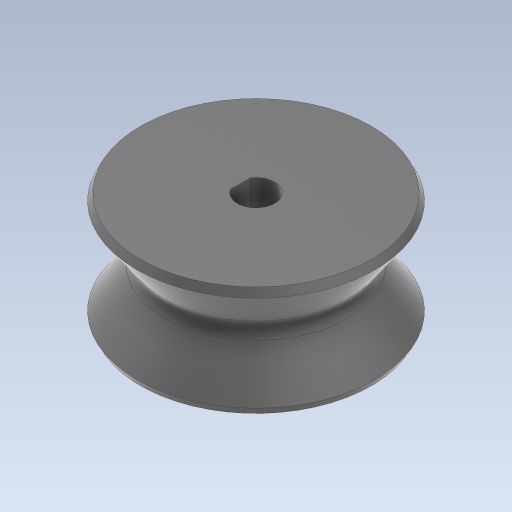
# Autodesk Inventor part: Stepper Pulley V12
Saved by Autodesk Inventor 2023 (Build 270158000, 158)
## iProperties
Created: 2022-07-02
Part Number: Stepper Pulley V12
Material: Thermoplastic Resin
Document SubType Name: Modeling
Designer: david
Density: 1.28 g/cm^3
Appearance: Smooth - Black
Author: david
## iProperties of the stored document Stepper Pulley V12_3DPrint.ipt
Created: 2022-11-09
Part Number: Stepper Pulley V12_3DPrint
Material: Generic
Document SubType Name: Modeling
Designer: Dave
Density: 1 g/cm^3
Appearance: Default
Author: Dave
Autodesk Inventor part; units mm, degrees
ref_plane "YZ Plane" through (0, 0, 0) normal (1, 0, 0) x (0, 1, 0)
sketch "Sketch1" plane through (0, 0, 0) normal (0, 1, 0) x (-1, 0, 0)
  arc A0 (2.15, 1.3711) -> (2.15, -1.3711) centre (0, 0) ccw
  line L0 (2.15, 1.3711) -> (2.15, -1.3711)
  dimension "d1" = 4.7
  dimension "d92" = 2.55
  constraints: 2 end point, 2 point on circle, 1 centre point, 1 coincident, 1 vertical
  measures "d92" radius of A0
sketch "Sketch2" plane through (0, 0, 0) normal (1, 0, 0) x (0, 1, 0)
  line L0 (0, 0) -> (15, 0)
  line L1 (15, 0) -> (15, -14)
  line L2 (0, 0) -> (0, -14)
  line L3 (5, -10) -> (15, -17.0021)
  line L4 (15, -14) -> (15, -17.0021)
  line L5 (7.5, 0) -> (7.5, -2.5713) construction
  line L6 (10, -10) -> (0, -17.0021)
  line L7 (0, -14) -> (0, -17.0021)
  point P0 (7.5, -11.7505)
  dimension "d4" = 15
  dimension "d5" = 14
  dimension "d6" = 14
  dimension "d93" = 10
  dimension "d102" = 55
  dimension "d103" = 10
  constraints: 16 end point, 4 vertical, 2 symmetric about line, 1 horizontal, 1 midpoint
  measures "d4" distance of L0.start L0.end
  measures "d5" distance of L0.end L1.end
  measures "d6" distance of L0.start L2.end
  measures "d93" distance from line of L1 L3.start
  measures "d102" angle of L2 L3
  measures "d103" distance from line of L0 L3.start
revolve "Revolution1" add sketch "Sketch2" angle 360 about axis through (0, 0, 0) along (0, 1, 0)
extrude "Extrusion1" cut sketch "Sketch1" along normal through all
chamfer "Chamfer1" distance 1.2 angle 45 2 edges at (0, 15, 17.0021) (0, 0, 17.0021)
ref_plane "Work Plane3" through (-14.15, 0, 1.3711) normal (1, 0, 0) x (0, 0, -1)
ref_plane "Work Plane4" through (0, 7.5, 0) normal (0, -1, 0) x (1, 0, 0)
fillet "Fillet1" radius 2 1 edges at (0, 7.5, 11.7505)
chamfer "Chamfer2" distance 1 angle 45 2 edges at (-2.15, 0, 0) (2.55, 0, 0)
hole "Hole4" at (0, 0, 0) direction (0, 1, 0) diameter 6.5 depth 5.3
chamfer "Chamfer3" distance 0.2 angle 45 3 edges at (-2.15, 5.3, 0) (2.55, 5.3, 0) (0, 5.3, 3.25)
equation "\"d6\" = d5"
body "Solid1"
